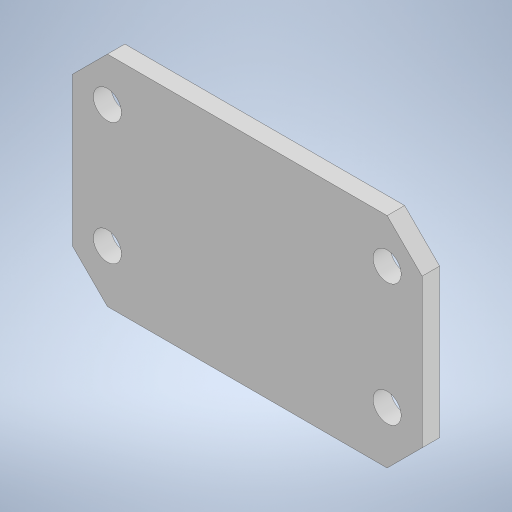
# Autodesk Inventor part: стена_простая
Saved by Autodesk Inventor 2023.1 (Build 271208000, 208)
## iProperties
Created: 2025-12-16
Part Number: стена_простая
Material: Типовые
Document SubType Name: Modeling
Designer: DELL
Density: 1 g/cm^3
Appearance: По умолчанию
Author: DELL
Autodesk Inventor part; units mm, degrees
ref_plane "YZ Plane" through (0, 0, 0) normal (1, 0, 0) x (0, 1, 0)
ref_plane "XZ Plane" through (0, 0, 0) normal (0, 1, 0) x (-1, 0, 0)
ref_plane "XY Plane" through (0, 0, 0) normal (0, 0, 1) x (1, 0, 0)
sketch "Эскиз1" plane through (0, 0, 0) normal (0, 0, 1) x (1, 0, 0)
  line L0 (-20.939, -15) -> (19.061, -15)
  line L1 (19.061, -15) -> (19.061, 10)
  line L2 (19.061, 10) -> (-20.939, 10)
  line L3 (-20.939, 10) -> (-20.939, -15)
  circle A0 centre (-16.939, 5) radius 1.6
  circle A1 centre (-16.939, -9) radius 1.6
  circle A2 centre (15.061, 5) radius 1.6
  circle A3 centre (15.061, -9) radius 1.6
  point P0 (0, 0)
  dimension "d0" = 40
  dimension "d5" = 3.2
  dimension "d7" = 14
  dimension "d16" = 3.2
  dimension "d17" = 3.2
  dimension "d18" = 3.2
  dimension "d19" = 5
  dimension "d20" = 14
  dimension "d21" = 6
  dimension "d22" = 6
  dimension "d23" = 4
  dimension "d25" = 4
  dimension "d26" = 4
  constraints: 8 end point, 4 centre point, 2 parallel, 1 horizontal, 1 perpendicular
  measures "d0" distance of L2.end L1.end
  measures "d5" diameter of A1
  measures "d7" distance of A1.centre A0.centre
  measures "d16" diameter of A2
  measures "d17" diameter of A3
  measures "d18" diameter of A0
  measures "d19" distance from line of L2 A2.centre
  measures "d20" distance of A3.centre A2.centre
  measures "d21" distance from line of L0 A3.centre
  measures "d22" distance from line of L0 A1.centre
  measures "d23" distance from line of L3 A1.centre
  measures "d25" distance from line of L3 A0.centre
  measures "d26" distance from line of L1 A2.centre
extrude "Выдавливание1" add sketch "Эскиз1" along normal blind 2
chamfer "Фаска1" distance 4 angle 45 4 edges at (19.061, 10, 1) (-20.939, 10, 1) (19.061, -15, 1) (-20.939, -15, 1)
